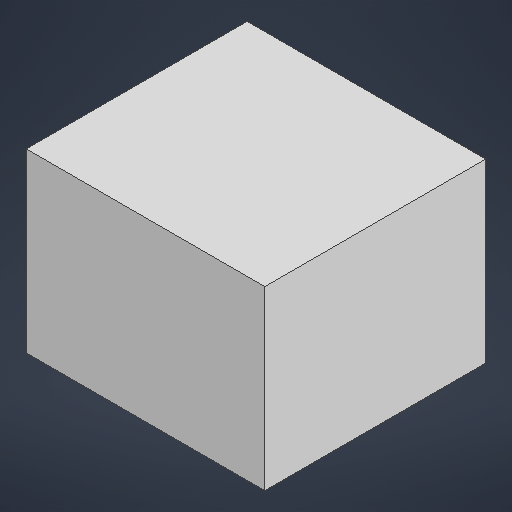
# Autodesk Inventor part: NI PXIe_1071
Saved by Autodesk Inventor 2026.2 (Build 302298010, 298A)
## iProperties
Created: 2026-09-21
Part Number: NI PXIe_1071
Material: Generic
Document SubType Name: Modeling
Designer: aiden
Density: 1 g/cm^3
Appearance: Default
Author: aiden
Autodesk Inventor part; units mm, degrees
ref_plane "YZ Plane" through (0, 0, 0) normal (1, 0, 0) x (0, 1, 0)
ref_plane "XZ Plane" through (0, 0, 0) normal (0, 1, 0) x (-1, 0, 0)
ref_plane "XY Plane" through (0, 0, 0) normal (0, 0, 1) x (1, 0, 0)
sketch "Sketch1" plane through (0, 0, 0) normal (0, 1, 0) x (-1, 0, 0)
  line L0 (-128.5875, -119.0625) -> (128.5875, -119.0625)
  line L1 (128.5875, -119.0625) -> (128.5875, 119.0625)
  line L2 (128.5875, 119.0625) -> (-128.5875, 119.0625)
  line L3 (-128.5875, 119.0625) -> (-128.5875, -119.0625)
  line L4 (-128.5875, -119.0625) -> (128.5875, 119.0625) construction
  line L5 (128.5875, -119.0625) -> (-128.5875, 119.0625) construction
  point P0 (0, 0)
  dimension "d0" = 257.175
  dimension "d1" = 238.125
  constraints: 12 end point, 2 midpoint, 2 parallel, 1 horizontal, 1 perpendicular
  measures "d0" distance of L2.end L1.end
  measures "d1" distance of L0.end L1.end
extrude "Extrusion1" add sketch "Sketch1" along normal blind 190.5
body "Solid1"
